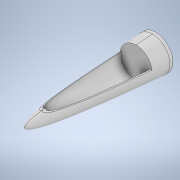
# Autodesk Inventor part: nose-basepart1
Saved by Autodesk Inventor 2020.3 (Build 243373000, 373)
## iProperties
Created: 2021-03-10
Part Number: nose-basepart1
Material: Generic
Document SubType Name: Modeling
Designer: 0x6f736f646f
Density: 1 g/cm^3
Appearance: Default
Author: 0x6f736f646f
Autodesk Inventor part; units mm, degrees
ref_plane "YZ Plane" through (0, 0, 0) normal (1, 0, 0) x (0, 1, 0)
ref_plane "XZ Plane" through (0, 0, 0) normal (0, 1, 0) x (-1, 0, 0)
ref_plane "XY Plane" through (0, 0, 0) normal (0, 0, 1) x (1, 0, 0)
sketch "Sketch1" plane through (0, 0, 0) normal (1, 0, 0) x (0, 1, 0)
  line L0 (0, 0) -> (25, 0)
  line L1 (25, 0) -> (25, -5)
  line L2 (25, -5) -> (26.8, -5)
  line L3 (26.8, -5) -> (26.8, 0)
  line L4 (0, 0) -> (0, 200)
  spline S0 degree 2 poles (26.8, 0) (13.4, 200) (0, 200) knots 0 0 0 0.5 0.5 0.5
  line L5 (1.9566, 200) -> (-1.9566, 200) construction
  arc A0 (1.1799, 199.5579) -> (-1.1799, 199.5579) centre (0, 198.2044) ccw construction
  line L6 (0, 160.0002) -> (11.7504, 160.0002) construction
  line L7 (0, 161.8) -> (13.7857, 161.8) construction
  spline S1 degree 2 poles (25, 0) (24.7387, 4.1433) (24.4774, 8.2) knots 0 0 0 1 1 1
  line L8 (24.5307, 7.3724) -> (24.4241, 9.0276) construction
  arc A1 (24.52, 7.5379) -> (24.4347, 8.8621) centre (-5899.3235, -373.3767) ccw construction
  line L9 (10.1029, 165.8331) -> (10.1029, 25.8331)
  line L10 (10.1029, 165.8331) -> (150.1029, 165.8331) construction
  line L11 (10.1029, 25.8331) -> (25.0094, 25.8331)
  line L12 (0, 170) -> (9.3945, 175.4239)
  line L13 (0, 170) -> (11.3645, 170) construction
  line L14 (0, 171.8) -> (8.2591, 176.5684)
  line L15 (0, 171.8) -> (0, 170)
  spline S2 degree 2 poles (24.4774, 8.2) (16.522, 131.7266) (8.5658, 174.9455) knots 0 0 0 1 1 1
  spline S3 degree 2 poles (8.2614, 176.5697) (4.1308, 198.2099) (0, 198.2044) knots 0 0 0 1 1 1
  line L16 (10.1897, 166.1244) -> (6.942, 183.7666) construction
  arc A2 (9.7692, 167.8737) -> (7.172, 181.9822) centre (-252.6717, 126.854) ccw construction
  line L17 (9.1499, 171.9152) -> (7.373, 181.2243) construction
  arc A3 (8.9426, 172.8409) -> (7.5213, 180.2873) centre (-226.6717, 131.7265) ccw construction
  line L18 (8.2591, 176.5684) -> (8.2614, 176.5697)
  line L19 (0, 24.0331) -> (23.4355, 24.0331)
  line L20 (0, 22.2331) -> (23.5563, 22.2331)
  line L21 (10.1029, 25.8331) -> (0, 25.8331)
  point P0 (-25, 0)
  point P1 (-26.8, 0)
  point P2 (0, 198.2)
  point P3 (0, 10)
  point P4 (0, 8.2)
  point P5 (24.3612, 10)
  point P6 (23.3141, 25.8331)
  dimension "d0" = 25
  dimension "d1" = 5
  dimension "d2" = 1.8
  dimension "d3" = 200
  dimension "d7" = 140
  dimension "d8" = 90
  dimension "d11" = 30
  dimension "d13" = 1.8
  dimension "d14" = 1.8
  constraints: 42 end point, 8 midpoint, 7 horizontal, 5 perpendicular, 4 centre point, 4 point on circle, 2 point on line, 2 vertical, 1 parallel, 32 other
  measures "d0" distance of L0.start L0.end
  measures "d1" distance of L0.end L1.end
  measures "d2" distance of L1.end L2.end
  measures "d3" distance of point (0, 200) L0.start
  measures "d7" distance of L9.start L9.end
  measures "d8" angle of L9 L10
  measures "d11" angle of L13 L12
  measures "d13" distance between parallel lines of L19 L11
  measures "d14" distance between parallel lines of L20 L19
revolve "Revolution1" add sketch "Sketch1" angle 360 about axis through (0, 0, 0) along (0, 0, 1) contours S1 S2 L11 S0 L3 L2 L1 | L4 L19 S2 L20 | L4 L21 L11 S2 L19 | L4 L14 L18 S3 S0 L12 | S2 L12 S0 L11
revolve "Revolution2" cut sketch "Sketch1" angle 210 mid plane about axis through (0, 10.1029, 165.8331) along (0, 0, -1) fills toward (10.1529, 95.8331) open curves L9 L11
body "Solid1"
